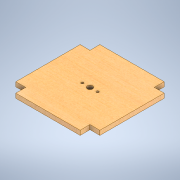
# Autodesk Inventor part: 上部3分木板中板
Saved by Autodesk Inventor 2021 (Build 250183000, 183)
## iProperties
Created: 2023-01-12
Part Number: 上部3分木板中板
Material: 松木、赤松
Document SubType Name: Modeling
Designer: brian
Density: 0.496 g/cm^3
Appearance: 黃色松木 - 深色中亮度
Author: brian
Autodesk Inventor part; units mm, degrees
ref_plane "YZ Plane" through (0, 0, 0) normal (1, 0, 0) x (0, 1, 0)
ref_plane "XZ Plane" through (0, 0, 0) normal (0, 1, 0) x (-1, 0, 0)
ref_plane "XY Plane" through (0, 0, 0) normal (0, 0, 1) x (1, 0, 0)
sketch "草圖1" plane through (0, 0, 0) normal (0, 1, 0) x (-1, 0, 0)
  line L0 (85, 85) -> (-85, 85)
  line L1 (-85, 85) -> (-85, -85)
  line L2 (-85, -85) -> (85, -85)
  line L3 (85, -85) -> (85, 85)
  line L4 (85, 85) -> (-85, -85) construction
  line L5 (-85, 85) -> (85, -85) construction
  point P0 (0, 0)
  dimension "d0" = 170
  dimension "d1" = 170
  constraints: 12 end point, 2 midpoint, 2 parallel, 1 horizontal, 1 perpendicular
  measures "d0" distance of L2.end L1.end
  measures "d1" distance of L1.end L0.end
extrude "擠出1" add sketch "草圖1" along normal blind 9
sketch "草圖2" plane through (0, 9, 0) normal (0, 1, 0) x (1, 0, 0)
  line L0 (-85, 85) -> (-85, -85) projected
  line L1 (-85, -85) -> (-65, -85)
  line L2 (-65, -85) -> (-65, -65)
  line L3 (-65, -65) -> (-85, -65)
  line L4 (-85, -65) -> (-85, -85)
  point P0 (0, 0)
  dimension "d4" = 20
  dimension "d5" = 20
  constraints: 8 end point, 2 parallel, 1 horizontal, 1 perpendicular
  measures "d4" distance of L3.end L2.end
  measures "d5" distance of L2.end L1.end
extrude "擠出2" cut sketch "草圖2" against normal through all
pattern_circular "環形陣列1" count 4 over 360 about axis through (0, -10, 0) along (0, 1, 0) of "擠出2"
sketch "草圖5" plane through (0, 9, 0) normal (0, 1, 0) x (1, 0, 0)
  point P0 (0, 0)
  point P1 (0, 0)
  constraints: 1 coincident
hole "孔3" at (0, 9, 0) direction (0, -1, 0) diameter 11 end through all
sketch "草圖6" plane through (0, 9, 0) normal (0, 1, 0) x (1, 0, 0)
  point P0 (0, 0)
  point P1 (-15.5, 0)
  point P2 (15.5, 0)
  dimension "d36" = 31
  dimension "d37" = 15.5
  constraints: 2 horizontal alignment
  measures "d36" distance of point (15.5, 0) point (-15.5, 0)
  measures "d37" distance of point (0, 0) point (15.5, 0)
hole "孔4" at (-15.5, 9, 0) at (15.5, 9, 0) direction (0, -1, 0) diameter 5 end through all
equation "\"d0\" = d1"
equation "\"d37\" = 0.5 * d36"
